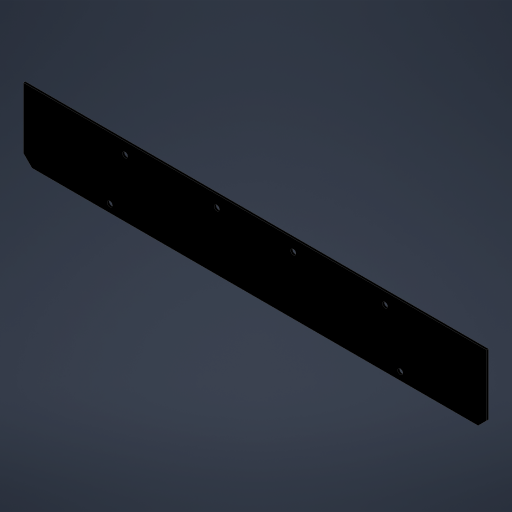
# Autodesk Inventor part: Back Guard
Saved by Autodesk Inventor 2023 (Build 270158000, 158)
## iProperties
Created: 2023-02-13
Part Number: Back Guard
Material: Generic
Document SubType Name: Modeling
Designer: alex
Density: 1 g/cm^3
Appearance: Default
Author: alex
Autodesk Inventor part; units mm, degrees
ref_plane "YZ Plane" through (0, 0, 0) normal (1, 0, 0) x (0, 1, 0)
ref_plane "XZ Plane" through (0, 0, 0) normal (0, 1, 0) x (-1, 0, 0)
ref_plane "XY Plane" through (0, 0, 0) normal (0, 0, 1) x (1, 0, 0)
sketch "Sketch1" plane through (0, 0, 0) normal (0, 0, 1) x (1, 0, 0)
  line L0 (84.4677, 12.3696) -> (-300.3677, 12.3696)
  line L1 (-300.3677, 12.3696) -> (-300.3677, -38.4304)
  line L2 (84.4677, -38.4304) -> (84.4677, 12.3696)
  circle A0 centre (0, 2.54) radius 2.1463
  line L3 (84.4677, -38.4304) -> (77.3473, -45.5508)
  line L4 (84.4677, -38.4304) -> (94.5374, -38.4304) construction
  line L5 (-300.3677, -38.4304) -> (-296.831, -38.4304) construction
  line L6 (-300.3677, -38.4304) -> (-293.2473, -45.5508)
  line L7 (-300.3677, -38.4304) -> (-290.298, -38.4304) construction
  line L8 (77.3473, -45.5508) -> (-293.2473, -45.5508)
  circle A1 centre (-215.9, 2.54) radius 2.1463
  circle A2 centre (12.7, -39.0652) radius 2.1463
  circle A3 centre (-228.6, -39.0652) radius 2.1463
  circle A4 centre (-76.2, 2.54) radius 2.1463
  circle A5 centre (-139.7, 2.54) radius 2.1463
  point P0 (0, 0)
  dimension "d0" = 384.8354
  dimension "d1" = 4.2926
  dimension "d2" = 84.4677
  dimension "d3" = 9.8296
  dimension "d4" = 135
  dimension "d5" = 7.1204
  dimension "d6" = 45
  dimension "d7" = 7.1204
  dimension "d8" = 4.2926
  dimension "d9" = 9.8296
  dimension "d10" = 215.9
  dimension "d13" = 4.2926
  dimension "d14" = 71.7677
  dimension "d17" = 51.4348
  dimension "d18" = 4.2926
  dimension "d19" = 51.4348
  dimension "d20" = 71.7677
  dimension "d21" = 50.8
  dimension "d22" = 4.2926
  dimension "d23" = 76.2
  dimension "d24" = 4.2926
  dimension "d25" = 76.2
  dimension "d26" = 9.8296
  dimension "d27" = 9.8296
  constraints: 18 end point, 6 centre point, 4 horizontal, 2 equal length, 1 parallel, 1 perpendicular
  measures "d0" distance between parallel lines of L1 L2
  measures "d1" diameter of A0
  measures "d2" distance from line of L2 A0.centre
  measures "d3" distance from line of L0 A0.centre
  measures "d4" angle of L3 L4
  measures "d5" horizontal distance of L2.start L3.end
  measures "d6" angle of L6 L7
  measures "d7" horizontal distance of L1.end L6.end
  measures "d8" diameter of A1
  measures "d9" distance from line of L0 A1.centre
  measures "d10" distance of A0.centre A1.centre
  measures "d13" diameter of A2
  measures "d14" distance from line of L2 A2.centre
  measures "d17" distance from line of L0 A2.centre
  measures "d18" diameter of A3
  measures "d19" distance from line of L0 A3.centre
  measures "d20" distance from line of L1 A3.centre
  measures "d21" distance of L2.start L0.start
  measures "d22" diameter of A4
  measures "d23" distance of A4.centre A0.centre
  measures "d24" diameter of A5
  measures "d25" distance between centres of A1 A5
  measures "d26" distance from line of L0 A5.centre
  measures "d27" distance from line of L0 A4.centre
extrude "Extrusion2" add sketch "Sketch1" along normal blind 1.5875
body "Solid2"
